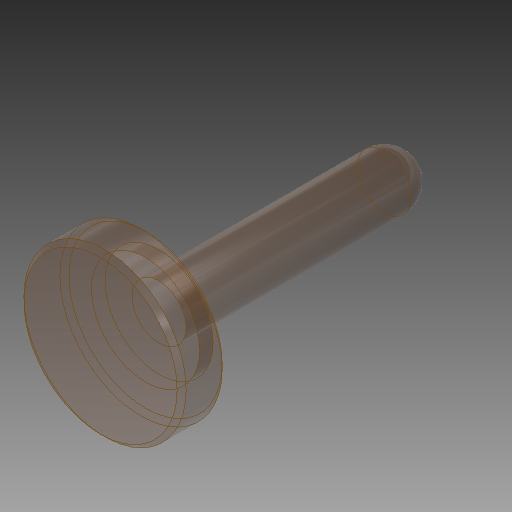
# Autodesk Inventor part: Pino de Liberação Valvula Alivio de Pressão
Saved by Autodesk Inventor 2019 (Build 230136000, 136)
## iProperties
Created: 2020-04-02
Part Number: Pino de Liberação Valvula Alivio de Pressão
Material: Genérico
Document SubType Name: Modeling
Designer: Paulo Rodrigues
Density: 1 g/cm^3
Appearance: Policarbonato - Fumê
Author: Paulo Rodrigues
Autodesk Inventor part; units mm, degrees
ref_plane "YZ Plane" through (0, 0, 0) normal (1, 0, 0) x (0, 1, 0)
ref_plane "XZ Plane" through (0, 0, 0) normal (0, 1, 0) x (-1, 0, 0)
ref_plane "XY Plane" through (0, 0, 0) normal (0, 0, 1) x (1, 0, 0)
sketch "Esboço1" plane through (0, 0, 0) normal (0, 0, 1) x (1, 0, 0)
  circle A0 centre (0, 0) radius 3.5 projected
  circle A1 centre (0, 0) radius 3
  point P0 (0, 0)
  dimension "d0" = 6
  constraints: 1 centre point, 1 coincident
  measures "d0" diameter of A1
extrude "Extrusão1" add sketch "Esboço1" against normal blind 25 contours A1
fillet "Arredondamento1" radius 3 1 edges at (-3, 0, -25)
sketch "Esboço2" plane through (0, 0, 0) normal (0, 0, 1) x (1, 0, 0)
  circle A0 centre (0, 0) radius 3 projected
  point P0 (0, 0)
extrude "Extrusão2" add sketch "Esboço2" along normal blind 3
sketch "Esboço3" plane through (0, 0, 3) normal (0, 0, 1) x (1, 0, 0)
  circle A0 centre (0, 0) radius 3 projected
  circle A1 centre (0, 0) radius 6
  point P0 (0, 0)
  dimension "d6" = 12
  constraints: 1 centre point, 1 coincident
  measures "d6" diameter of A1
extrude "Extrusão3" add sketch "Esboço3" along normal blind 1.5 contours A0 | A1
sketch "Esboço4" plane through (0, 0, 4.5) normal (0, 0, 1) x (1, 0, 0)
  circle A0 centre (0, 0) radius 9
  dimension "d9" = 18
  constraints: 1 centre point, 1 coincident
  measures "d9" diameter of A0
extrude "Extrusão4" add sketch "Esboço4" along normal blind 5
chamfer "Chanfro1" distance 0.5 angle 45 2 edges at (-9, 0, 9.5) (-9, 0, 4.5)
